Autodesk Fusion 360 part; units mm, degrees
note: some values were not read from the file. Chosen so that the rebuilt part matches the saved one: which face or edge a step refers to.
(part 2 of 2)
sketch "Sketch34" plane through (0, 0, 180) normal (0, 0, 1) x (-1, 0, 0)
  circle A0 centre (10, -110) radius 5
  line L0 (7, -103) -> (162.9875, -103)
  line L1 (166.9875, -107) -> (166.9875, -113)
  line L2 (162.9875, -117) -> (7, -117)
  line L3 (3, -113) -> (3, -107)
  arc A1 (7, -103) -> (3, -107) centre (7, -107) ccw
  arc A2 (166.9875, -107) -> (162.9875, -103) centre (162.9875, -107) ccw
  arc A3 (3, -113) -> (7, -117) centre (7, -113) ccw
  arc A4 (162.9875, -117) -> (166.9875, -113) centre (162.9875, -113) ccw
  line L4 (25, -115) -> (45, -115)
  line L5 (45, -115) -> (45, -3.8464)
  line L6 (41, 0.1536) -> (29, 0.1536)
  line L7 (25, -3.8464) -> (25, -115)
  arc A5 (29, 0.1536) -> (25, -3.8464) centre (29, -3.8464) ccw
  arc A6 (45, -3.8464) -> (41, 0.1536) centre (41, -3.8464) ccw
  line L8 (75, -3.8464) -> (75, -115)
  line L9 (95, -115) -> (95, -3.8464)
  line L10 (91, 0.1536) -> (79, 0.1536)
  arc A7 (95, -3.8464) -> (91, 0.1536) centre (91, -3.8464) ccw
  arc A8 (79, 0.1536) -> (75, -3.8464) centre (79, -3.8464) ccw
  line L11 (75, -115) -> (95, -115)
  line L12 (125, -3.8464) -> (125, -115)
  line L13 (145, -115) -> (145, -3.8464)
  line L14 (141, 0.1536) -> (129, 0.1536)
  arc A9 (145, -3.8464) -> (141, 0.1536) centre (141, -3.8464) ccw
  arc A10 (129, 0.1536) -> (125, -3.8464) centre (129, -3.8464) ccw
  line L15 (125, -115) -> (145, -115)
  dimension "d116" = 4
  dimension "d117" = 4
  dimension "d118" = 4
  dimension "d119" = 4
  dimension "d120" = 4
  dimension "d121" = 4
  dimension "d122" = 4
  dimension "d123" = 4
  dimension "d124" = 4
  dimension "d125" = 4
  constraint horizontal L0
  constraint vertical L1
  constraint horizontal L2
  constraint vertical L3
  constraint tangent L0 A1
  constraint tangent L3 A1
  constraint tangent L0 A2
  constraint tangent L1 A2
  constraint tangent L3 A3
  constraint tangent L2 A3
  constraint tangent L1 A4
  constraint tangent L2 A4
  constraint horizontal L4
  constraint vertical L5
  constraint horizontal L6
  constraint vertical L7
  constraint tangent L6 A5
  constraint tangent L7 A5
  constraint tangent L5 A6
  constraint tangent L6 A6
  constraint horizontal L11
  constraint vertical L9
  constraint horizontal L10
  constraint vertical L8
  constraint tangent L10 A8
  constraint tangent L8 A8
  constraint tangent L9 A7
  constraint tangent L10 A7
  constraint horizontal L15
  constraint vertical L13
  constraint horizontal L14
  constraint vertical L12
  constraint tangent L14 A10
  constraint tangent L12 A10
  constraint tangent L13 A9
  constraint tangent L14 A9
  measures "d116" radius of A1
  measures "d117" radius of A2
  measures "d118" radius of A3
  measures "d119" radius of A4
  measures "d120" radius of A5
  measures "d121" radius of A6
  measures "d122" radius of A8
  measures "d123" radius of A7
  measures "d124" radius of A10
  measures "d125" radius of A9
extrude "Extrude29" add sketch "Sketch34" along normal blind 5 bodies 12 11
sketch "Sketch35" plane through (0, 0, 185) normal (0, 0, 1) x (-1, 0, 0)
  circle A0 centre (10, -110) radius 5
  line L0 (145, -103) -> (145, -3.8464)
  arc A1 (145, -3.8464) -> (141, 0.1536) centre (141, -3.8464) ccw
  line L1 (141, 0.1536) -> (129, 0.1536)
  arc A2 (129, 0.1536) -> (125, -3.8464) centre (129, -3.8464) ccw
  line L2 (125, -3.8464) -> (125, -103)
  line L3 (125, -103) -> (95, -103)
  line L4 (95, -103) -> (95, -3.8464)
  arc A3 (95, -3.8464) -> (91, 0.1536) centre (91, -3.8464) ccw
  line L5 (91, 0.1536) -> (79, 0.1536)
  arc A4 (79, 0.1536) -> (75, -3.8464) centre (79, -3.8464) ccw
  line L6 (75, -3.8464) -> (75, -103)
  line L7 (75, -103) -> (45, -103)
  line L8 (45, -103) -> (45, -3.8464)
  arc A5 (45, -3.8464) -> (41, 0.1536) centre (41, -3.8464) ccw
  line L9 (41, 0.1536) -> (29, 0.1536)
  arc A6 (29, 0.1536) -> (25, -3.8464) centre (29, -3.8464) ccw
  line L10 (25, -3.8464) -> (25, -103)
  line L11 (25, -103) -> (7, -103)
  arc A7 (7, -103) -> (3, -107) centre (7, -107) ccw
  line L12 (3, -107) -> (3, -113)
  arc A8 (3, -113) -> (7, -117) centre (7, -113) ccw
  line L13 (7, -117) -> (162.9875, -117)
  arc A9 (162.9875, -117) -> (166.9875, -113) centre (162.9875, -113) ccw
  line L14 (166.9875, -113) -> (166.9875, -107)
  arc A10 (166.9875, -107) -> (162.9875, -103) centre (162.9875, -107) ccw
  line L15 (162.9875, -103) -> (145, -103)
  circle A11 centre (160, -110) radius 5
  dimension "d128" = 10
  measures "d128" diameter of A11
extrude "Extrude30" cut sketch "Sketch35" against normal blind 5 contours A11 bodies 12
sketch "Sketch36" plane through (0, 0, 180) normal (0, 0, -1) x (1, 0, 0)
  line L0 (-145, -3.8464) -> (-145, -103)
  line L1 (-145, -103) -> (-162.9875, -103)
  arc A0 (-162.9875, -103) -> (-166.9875, -107) centre (-162.9875, -107) ccw
  line L2 (-166.9875, -107) -> (-166.9875, -113)
  arc A1 (-166.9875, -113) -> (-162.9875, -117) centre (-162.9875, -113) ccw
  line L3 (-162.9875, -117) -> (-7, -117)
  arc A2 (-7, -117) -> (-3, -113) centre (-7, -113) ccw
  line L4 (-3, -113) -> (-3, -107)
  arc A3 (-3, -107) -> (-7, -103) centre (-7, -107) ccw
  line L5 (-7, -103) -> (-25, -103)
  line L6 (-25, -103) -> (-25, -3.8464)
  arc A4 (-25, -3.8464) -> (-29, 0.1536) centre (-29, -3.8464) ccw
  line L7 (-29, 0.1536) -> (-41, 0.1536)
  arc A5 (-41, 0.1536) -> (-45, -3.8464) centre (-41, -3.8464) ccw
  line L8 (-45, -3.8464) -> (-45, -103)
  line L9 (-45, -103) -> (-75, -103)
  line L10 (-75, -103) -> (-75, -3.8464)
  arc A6 (-75, -3.8464) -> (-79, 0.1536) centre (-79, -3.8464) ccw
  line L11 (-79, 0.1536) -> (-91, 0.1536)
  arc A7 (-91, 0.1536) -> (-95, -3.8464) centre (-91, -3.8464) ccw
  line L12 (-95, -3.8464) -> (-95, -103)
  line L13 (-95, -103) -> (-125, -103)
  line L14 (-125, -103) -> (-125, -3.8464)
  arc A8 (-125, -3.8464) -> (-129, 0.1536) centre (-129, -3.8464) ccw
  line L15 (-129, 0.1536) -> (-141, 0.1536)
  arc A9 (-141, 0.1536) -> (-145, -3.8464) centre (-141, -3.8464) ccw
  circle A10 centre (-10, -110) radius 5
  circle A11 centre (-160, -110) radius 5
  circle A12 centre (-135, -25) radius 4
  circle A13 centre (-85, -25) radius 4
  circle A14 centre (-35, -25) radius 4
  dimension "d131" = 8
  dimension "d132" = 8
  dimension "d133" = 8
  measures "d131" diameter of A12
  measures "d132" diameter of A13
  measures "d133" diameter of A14
extrude "Extrude31" add sketch "Sketch36" along normal blind 7 separate body contours A12 | A13 | A14 makes body 13 at (-137.7929, 22.1365, 175.3333) makes body 14 at (-81.0199, 25.3983, 175.3333) makes body 15 at (-31.0199, 25.3983, 175.3333)
extrude "Extrude32" add 2 faces at (-11.5202, 110.9715, 180) (-161.0391, 111.7999, 180) along direction (0, 0, 1) blind 100 on bodies 12 bodies 12
move_body "Move9" bodies 2 to x (1, 0, 0) y (0, 1, 0) z (0, 0, 1) at (-10, 0, 0)
copy_body "CopyPasteBodies2" bodies 2 makes body 16
move_body "Move11" bodies 16 to x (1, 0, 0) y (0, 1, 0) z (0, 0, 1) at (-52, 0, 0)
copy_body "CopyPasteBodies3" bodies 16 makes body 17
move_body "Move12" bodies 17 to x (1, 0, 0) y (0, 1, 0) z (0, 0, 1) at (-52, 0, 0)
component "Component" placed x (1, 0, 0) y (0, 1, 0) z (0, 0, 1) at (0, 0, 0)
